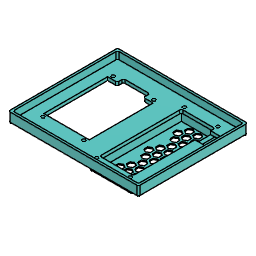
orient-beetle-screen-case-v2 v14 (Autodesk Fusion 360 design; units mm, degrees)
Autodesk Fusion 360 part; units mm, degrees
sketch "base-sketch" plane through (0, 0, 0) normal (0, 0, 1) x (1, 0, 0)
  line L0 (0, 0) -> (120, 0)
  line L1 (120, 0) -> (120, 100)
  line L2 (120, 100) -> (0, 100)
  line L3 (0, 100) -> (0, 0)
  line L4 (10, 19.5) -> (53.5, 19.5)
  line L5 (53.5, 19.5) -> (53.5, 80.5)
  line L6 (53.5, 80.5) -> (10, 80.5)
  line L7 (10, 80.5) -> (10, 19.5)
  line L8 (104, 11) -> (72, 11)
  line L9 (72, 11) -> (72, 89)
  line L10 (72, 89) -> (104, 89)
  line L11 (104, 89) -> (104, 11)
  line L12 (44.25, 86.5) -> (19.25, 86.5)
  line L13 (19.25, 86.5) -> (19.25, 80.5)
  line L14 (19.25, 80.5) -> (44.25, 80.5)
  line L15 (44.25, 80.5) -> (44.25, 86.5)
  line L16 (31.75, 19.5) -> (31.75, 80.5) construction
  line L17 (31.75, 80.5) -> (31.75, 86.5) construction
  line L18 (104, 70) -> (114, 70)
  line L19 (114, 70) -> (114, 85)
  line L20 (114, 85) -> (104, 85)
  line L21 (104, 85) -> (104, 70)
  circle A0 centre (116, 72.5) radius 1.25
  circle A1 centre (116, 82.5) radius 1.25
  line L22 (116, 72.5) -> (116, 82.5) construction
  line L23 (104, 77.5) -> (114, 77.5)
  circle A2 centre (12.25, 16.5) radius 1.6
  line L24 (10, 50) -> (53.5, 50) construction
  circle A3 centre (51.25, 16.5) radius 1.6
  circle A4 centre (12.25, 83.5) radius 1.6
  circle A5 centre (51.25, 83.5) radius 1.6
  line L25 (122.1, 102.1) -> (-2.1, 102.1)
  line L26 (-2.1, 102.1) -> (-2.1, -2.1)
  line L27 (-2.1, -2.1) -> (122.1, -2.1)
  line L28 (122.1, -2.1) -> (122.1, 102.1)
  point P0 (116, 77.5)
  dimension "d1" = 120
  dimension "d2" = 100
  dimension "d3" = 43.5
  dimension "d4" = 61
  dimension "d6" = 10
  dimension "d7" = 32
  dimension "d8" = 78
  dimension "d9" = 16
  dimension "d10" = 11
  dimension "d11" = 19.5
  dimension "d12" = 19.5
  dimension "d13" = 11
  dimension "d14" = 25
  dimension "d15" = 6
  dimension "d20" = 10
  dimension "d21" = 15
  dimension "d22" = 15
  dimension "d23" = 2.5
  dimension "d24" = 2.5
  dimension "d25" = 10
  dimension "d27" = 12
  dimension "d28" = 3.2
  dimension "d31" = 3.2
  dimension "d33" = 3.2
  dimension "d40" = 19.5
  dimension "d41" = 33.5
  dimension "d42" = 3.2
  dimension "d43" = 39
  dimension "d44" = 33.5
  dimension "d45" = 33.5
  dimension "d46" = 33.5
  dimension "d47" = 39
  dimension "d48" = 19.5
  dimension "d49" = 2.1
  constraint horizontal L0
  constraint vertical L1
  constraint horizontal L2
  constraint vertical L3
  constraint coincident L0.start L3.end
  constraint horizontal L4
  constraint vertical L5
  constraint horizontal L6
  constraint vertical L7
  constraint horizontal L8
  constraint vertical L9
  constraint horizontal L10
  constraint vertical L11
  constraint horizontal L12
  constraint vertical L13
  constraint horizontal L14
  constraint vertical L15
  constraint midpoint L4 L16.start
  constraint midpoint L6 L16.end
  constraint midpoint L14 L16.end
  constraint midpoint L12 L17.end
  constraint collinear L16 L17
  constraint collinear L6 L14
  constraint horizontal L18
  constraint vertical L19
  constraint horizontal L20
  constraint vertical L21
  constraint collinear L11 L21
  constraint coincident A0.centre L22.start
  constraint coincident A1.centre L22.end
  constraint parallel L19 L22
  constraint midpoint L21 L23.start
  constraint midpoint L19 L23.end
  constraint midpoint L22 P0
  constraint coincident L23 P0
  constraint midpoint L7 L24.start
  constraint midpoint L5 L24.end
  measures "d1" distance of L0.start L0.end
  measures "d2" distance of L0.start L2.end
  measures "d3" distance of L4.start L4.end
  measures "d4" distance of L4.start L6.end
  measures "d6" distance of L3 L7
  measures "d7" distance of L8.start L8.end
  measures "d8" distance of L8.start L10.end
  measures "d9" distance of L1 L11
  measures "d10" distance of L0 L8
  measures "d11" distance of L2 L6
  measures "d12" distance of L0 L4
  measures "d13" distance of L2 L10
  measures "d14" distance of L12.start L12.end
  measures "d15" distance of L12.end L13.end
  measures "d20" distance of L19.end L20.end
  measures "d21" distance of L18.end L19.end
  measures "d22" distance of L2 L20
  measures "d23" diameter of A0
  measures "d24" diameter of A1
  measures "d25" distance of A0.centre A1.centre
  measures "d27" distance of L21 A0.centre
  measures "d28" diameter of A2
  measures "d31" diameter of A3
  measures "d33" diameter of A4
  measures "d40" distance of L16 A4.centre
  measures "d41" distance of L24 A4.centre
  measures "d42" diameter of A5
  measures "d43" distance of A4.centre A5.centre
  measures "d44" distance of L24 A5.centre
  measures "d45" distance of A2.centre L24
  measures "d46" distance of L24 A3.centre
  measures "d47" distance of A2.centre A3.centre
  measures "d48" distance of L16 A2.centre
sketch "beetle-expansion" plane through (0, 0, 0) normal (0, 0, 1) x (1, 0, 0)
  line L0 (72, 89) -> (104, 89)
  line L1 (104, 89) -> (104, 11)
  line L2 (104, 11) -> (72, 11)
  line L3 (72, 11) -> (72, 89)
  line L4 (68, 7) -> (68, 93)
  line L5 (68, 93) -> (108, 93)
  line L6 (108, 93) -> (108, 7)
  line L7 (108, 7) -> (68, 7)
  dimension "d60" = -4
extrude "Extrude3" add sketch "beetle-expansion" against normal blind 8 makes body 1
sketch "beetle-expansion-top" plane through (0, 0, -8) normal (0, 0, -1) x (1, 0, 0)
  line L0 (72, -11) -> (104, -11)
  line L1 (104, -11) -> (104, -89)
  line L2 (104, -89) -> (72, -89)
  line L3 (72, -89) -> (72, -11)
  line L4 (108, -93) -> (108, -7)
  line L5 (108, -7) -> (68, -7)
  line L6 (68, -7) -> (68, -93)
  line L7 (68, -93) -> (108, -93)
  line L8 (104, -11) -> (104, -89)
  line L9 (72, -11) -> (104, -11)
  line L10 (72, -89) -> (72, -11)
  line L11 (104, -89) -> (72, -89)
extrude "Extrude1" add sketch "base-sketch" along normal blind 3.2 separate body contours L0 L1 L2 L3 makes body 2
extrude "Extrude2" add sketch "base-sketch" along normal blind 10 contours L25 L26 L27 L28 bodies 2
fillet "Fillet1" radius 1.5 8 edges at (-2.1, 102.1, 5) (122.1, 102.1, 5) (120, 0, 6.6) (-2.1, -2.1, 5) (0, 0, 6.6) (0, 100, 6.6) (120, 100, 6.6) (122.1, -2.1, 5) on bodies 2
fillet "Fillet2" radius 1.5 6 edges at (104, 11, 1.6) (72, 11, 1.6) (72, 89, 1.6) (104, 89, 1.6) (114, 70, 1.6) (114, 85, 1.6) on bodies 2
fillet "Fillet3" radius 1.5 2 edges at (44.25, 86.5, 1.6) (19.25, 86.5, 1.6) on bodies 2
extrude "Extrude6" add sketch "beetle-expansion-top" against normal blind 1 contours L0 L1 L2 L3 L8 L9 L10 L11 bodies 1
move_face "OffsetFaces1" offset 2 2 faces at (81.3333, 93, -5.3333) (94.6667, 7, -5.3333) on bodies 1
sketch "expansion-holes" plane through (0, 0, 3.2) normal (0, 0, 1) x (-1, 0, 0)
  line L0 (-44.25, -85) -> (-44.25, -80.5)
  line L1 (-44.25, -80.5) -> (-53.5, -80.5)
  line L2 (-53.5, -80.5) -> (-53.5, -19.5)
  line L3 (-53.5, -19.5) -> (-10, -19.5)
  line L4 (-10, -19.5) -> (-10, -80.5)
  line L5 (-10, -80.5) -> (-19.25, -80.5)
  line L6 (-19.25, -80.5) -> (-19.25, -85)
  arc A0 (-20.75, -86.5) -> (-19.25, -85) centre (-20.75, -85) ccw
  line L7 (-20.75, -86.5) -> (-42.75, -86.5)
  arc A1 (-44.25, -85) -> (-42.75, -86.5) centre (-42.75, -85) ccw
  line L8 (-112.5, -70) -> (-104, -70)
  line L9 (-104, -70) -> (-104, -12.5)
  arc A2 (-102.5, -11) -> (-104, -12.5) centre (-102.5, -12.5) ccw
  line L10 (-102.5, -11) -> (-73.5, -11)
  arc A3 (-72, -12.5) -> (-73.5, -11) centre (-73.5, -12.5) ccw
  line L11 (-72, -12.5) -> (-72, -87.5)
  arc A4 (-73.5, -89) -> (-72, -87.5) centre (-73.5, -87.5) ccw
  line L12 (-73.5, -89) -> (-102.5, -89)
  arc A5 (-104, -87.5) -> (-102.5, -89) centre (-102.5, -87.5) ccw
  line L13 (-104, -87.5) -> (-104, -85)
  line L14 (-104, -85) -> (-112.5, -85)
  arc A6 (-114, -83.5) -> (-112.5, -85) centre (-112.5, -83.5) ccw
  line L15 (-114, -83.5) -> (-114, -71.5)
  arc A7 (-112.5, -70) -> (-114, -71.5) centre (-112.5, -71.5) ccw
  circle A8 centre (-116, -82.5) radius 1.25
  circle A9 centre (-116, -72.5) radius 1.25
  circle A10 centre (-51.25, -83.5) radius 1.6
  circle A11 centre (-12.25, -83.5) radius 1.6
  circle A12 centre (-51.25, -16.5) radius 1.6
  circle A13 centre (-12.25, -16.5) radius 1.6
  arc A14 (-120, -98.5) -> (-118.5, -100) centre (-118.5, -98.5) ccw
  line L16 (-118.5, -100) -> (-1.5, -100)
  arc A15 (-1.5, -100) -> (0, -98.5) centre (-1.5, -98.5) ccw
  line L17 (0, -98.5) -> (0, -1.5)
  arc A16 (0, -1.5) -> (-1.5, 0) centre (-1.5, -1.5) ccw
  line L18 (-1.5, 0) -> (-118.5, 0)
  arc A17 (-118.5, 0) -> (-120, -1.5) centre (-118.5, -1.5) ccw
  line L19 (-120, -1.5) -> (-120, -98.5)
  circle A18 centre (-72, -92) radius 1.6
  line L20 (-68, -93) -> (-108, -93)
  line L21 (-68, -7) -> (-68, -93)
  line L22 (-72, -89) -> (-104, -89)
  dimension "d88" = 4
  dimension "d89" = 3.2
  dimension "d96" = 3
  measures "d88" distance of A18.centre L21
  measures "d89" diameter of A18
  measures "d96" distance of A18.centre L22
extrude "Extrude7" cut sketch "expansion-holes" against normal blind 15 contours A18 L20 | A18 L20 bodies 1 2
pattern_linear "R-Pattern1" count 2 spacing 32 along (1, 0, 0) count 2 spacing 84 along (0, -1, 0) of "Extrude7"
fillet "Fillet5" radius 1.5 4 edges at (68, 95, -4) (108, 95, -4) (68, 5, -4) (108, 5, -4) on bodies 1
sketch "honeycomb" plane through (0, 0, -8) normal (0, 0, -1) x (1, 0, 0)
  line L0 (104, -11) -> (72, -11) construction
  line L1 (72, -11) -> (72, -89) construction
  line L2 (104, -89) -> (104, -11) construction
  line L3 (72, -89) -> (104, -89) construction
  line L4 (104, -50) -> (72, -50) construction
  line L5 (88, -11) -> (88, -89) construction
  line L6 (88, -53.4641) -> (91, -51.7321)
  line L7 (91, -51.7321) -> (91, -48.2679)
  line L8 (91, -48.2679) -> (88, -46.5359)
  line L9 (88, -46.5359) -> (85, -48.2679)
  line L10 (85, -48.2679) -> (85, -51.7321)
  line L11 (85, -51.7321) -> (88, -53.4641)
  line L12 (88, -50) -> (86.5, -52.5981) construction
  line L13 (86.5, -52.5981) -> (86, -53.4641) construction
  line L14 (88, -50) -> (89.5, -52.5981) construction
  line L15 (84, -46.5359) -> (87, -44.8038)
  line L16 (87, -44.8038) -> (87, -41.3397)
  line L17 (87, -41.3397) -> (84, -39.6077)
  line L18 (84, -39.6077) -> (81, -41.3397)
  line L19 (81, -44.8038) -> (84, -46.5359)
  line L20 (81, -41.3397) -> (81, -44.8038)
  line L21 (80, -53.4641) -> (83, -51.7321)
  line L22 (83, -51.7321) -> (83, -48.2679)
  line L23 (83, -48.2679) -> (80, -46.5359)
  line L24 (80, -46.5359) -> (77, -48.2679)
  line L25 (77, -51.7321) -> (80, -53.4641)
  line L26 (77, -48.2679) -> (77, -51.7321)
  line L27 (92, -46.5359) -> (95, -44.8038)
  line L28 (95, -44.8038) -> (95, -41.3397)
  line L29 (95, -41.3397) -> (92, -39.6077)
  line L30 (92, -39.6077) -> (89, -41.3397)
  line L31 (89, -44.8038) -> (92, -46.5359)
  line L32 (89, -41.3397) -> (89, -44.8038)
  line L33 (84, -60.3923) -> (87, -58.6603)
  line L34 (87, -58.6603) -> (87, -55.1962)
  line L35 (87, -55.1962) -> (84, -53.4641)
  line L36 (84, -53.4641) -> (81, -55.1962)
  line L37 (81, -58.6603) -> (84, -60.3923)
  line L38 (81, -55.1962) -> (81, -58.6603)
  line L39 (96, -53.4641) -> (99, -51.7321)
  line L40 (99, -51.7321) -> (99, -48.2679)
  line L41 (99, -48.2679) -> (96, -46.5359)
  line L42 (96, -46.5359) -> (93, -48.2679)
  line L43 (93, -51.7321) -> (96, -53.4641)
  line L44 (93, -48.2679) -> (93, -51.7321)
  line L45 (92, -60.3923) -> (95, -58.6603)
  line L46 (95, -58.6603) -> (95, -55.1962)
  line L47 (95, -55.1962) -> (92, -53.4641)
  line L48 (92, -53.4641) -> (89, -55.1962)
  line L49 (89, -58.6603) -> (92, -60.3923)
  line L50 (89, -55.1962) -> (89, -58.6603)
  line L51 (87, -27.4962) -> (84, -25.7641)
  line L52 (84, -25.7641) -> (81, -27.4962)
  line L53 (81, -27.4962) -> (81, -30.9603)
  line L54 (81, -30.9603) -> (84, -32.6923)
  line L55 (87, -30.9603) -> (87, -27.4962)
  line L56 (84, -32.6923) -> (87, -30.9603)
  line L57 (95, -27.4962) -> (92, -25.7641)
  line L58 (92, -25.7641) -> (89, -27.4962)
  line L59 (89, -27.4962) -> (89, -30.9603)
  line L60 (89, -30.9603) -> (92, -32.6923)
  line L61 (95, -30.9603) -> (95, -27.4962)
  line L62 (92, -32.6923) -> (95, -30.9603)
  line L63 (99, -20.5679) -> (96, -18.8359)
  line L64 (96, -18.8359) -> (93, -20.5679)
  line L65 (93, -20.5679) -> (93, -24.0321)
  line L66 (93, -24.0321) -> (96, -25.7641)
  line L67 (99, -24.0321) -> (99, -20.5679)
  line L68 (96, -25.7641) -> (99, -24.0321)
  line L69 (95, -13.6397) -> (92, -11.9077)
  line L70 (92, -11.9077) -> (89, -13.6397)
  line L71 (89, -13.6397) -> (89, -17.1038)
  line L72 (89, -17.1038) -> (92, -18.8359)
  line L73 (95, -17.1038) -> (95, -13.6397)
  line L74 (92, -18.8359) -> (95, -17.1038)
  line L75 (81, -13.6397) -> (81, -17.1038)
  line L76 (81, -17.1038) -> (84, -18.8359)
  line L77 (84, -18.8359) -> (87, -17.1038)
  line L78 (87, -17.1038) -> (87, -13.6397)
  line L79 (84, -11.9077) -> (81, -13.6397)
  line L80 (87, -13.6397) -> (84, -11.9077)
  line L81 (77, -20.5679) -> (77, -24.0321)
  line L82 (77, -24.0321) -> (80, -25.7641)
  line L83 (80, -25.7641) -> (83, -24.0321)
  line L84 (83, -24.0321) -> (83, -20.5679)
  line L85 (80, -18.8359) -> (77, -20.5679)
  line L86 (83, -20.5679) -> (80, -18.8359)
  line L87 (85, -24.0321) -> (88, -25.7641)
  line L88 (88, -25.7641) -> (91, -24.0321)
  line L89 (91, -24.0321) -> (91, -20.5679)
  line L90 (91, -20.5679) -> (88, -18.8359)
  line L91 (85, -20.5679) -> (85, -24.0321)
  line L92 (88, -18.8359) -> (85, -20.5679)
  line L93 (87, -82.8962) -> (84, -81.1641)
  line L94 (84, -81.1641) -> (81, -82.8962)
  line L95 (81, -82.8962) -> (81, -86.3603)
  line L96 (81, -86.3603) -> (84, -88.0923)
  line L97 (87, -86.3603) -> (87, -82.8962)
  line L98 (84, -88.0923) -> (87, -86.3603)
  line L99 (95, -82.8962) -> (92, -81.1641)
  line L100 (92, -81.1641) -> (89, -82.8962)
  line L101 (89, -82.8962) -> (89, -86.3603)
  line L102 (89, -86.3603) -> (92, -88.0923)
  line L103 (95, -86.3603) -> (95, -82.8962)
  line L104 (92, -88.0923) -> (95, -86.3603)
  line L105 (99, -75.9679) -> (96, -74.2359)
  line L106 (96, -74.2359) -> (93, -75.9679)
  line L107 (93, -75.9679) -> (93, -79.4321)
  line L108 (93, -79.4321) -> (96, -81.1641)
  line L109 (99, -79.4321) -> (99, -75.9679)
  line L110 (96, -81.1641) -> (99, -79.4321)
  line L111 (95, -69.0397) -> (92, -67.3077)
  line L112 (92, -67.3077) -> (89, -69.0397)
  line L113 (89, -69.0397) -> (89, -72.5038)
  line L114 (89, -72.5038) -> (92, -74.2359)
  line L115 (95, -72.5038) -> (95, -69.0397)
  line L116 (92, -74.2359) -> (95, -72.5038)
  line L117 (81, -69.0397) -> (81, -72.5038)
  line L118 (81, -72.5038) -> (84, -74.2359)
  line L119 (84, -74.2359) -> (87, -72.5038)
  line L120 (87, -72.5038) -> (87, -69.0397)
  line L121 (84, -67.3077) -> (81, -69.0397)
  line L122 (87, -69.0397) -> (84, -67.3077)
  line L123 (77, -75.9679) -> (77, -79.4321)
  line L124 (77, -79.4321) -> (80, -81.1641)
  line L125 (80, -81.1641) -> (83, -79.4321)
  line L126 (83, -79.4321) -> (83, -75.9679)
  line L127 (80, -74.2359) -> (77, -75.9679)
  line L128 (83, -75.9679) -> (80, -74.2359)
  line L129 (85, -79.4321) -> (88, -81.1641)
  line L130 (88, -81.1641) -> (91, -79.4321)
  line L131 (91, -79.4321) -> (91, -75.9679)
  line L132 (91, -75.9679) -> (88, -74.2359)
  line L133 (85, -75.9679) -> (85, -79.4321)
  line L134 (88, -74.2359) -> (85, -75.9679)
  line L135 (91, -37.8771) -> (91, -34.4129)
  line L136 (91, -34.4129) -> (88, -32.6809)
  line L137 (88, -32.6809) -> (85, -34.4129)
  line L138 (85, -34.4129) -> (85, -37.8771)
  line L139 (88, -39.6091) -> (91, -37.8771)
  line L140 (85, -37.8771) -> (88, -39.6091)
  line L141 (91, -65.5871) -> (91, -62.1229)
  line L142 (91, -62.1229) -> (88, -60.3909)
  line L143 (88, -60.3909) -> (85, -62.1229)
  line L144 (85, -62.1229) -> (85, -65.5871)
  line L145 (88, -67.3191) -> (91, -65.5871)
  line L146 (85, -65.5871) -> (88, -67.3191)
  point P0 (88, -50)
  point P1 (88, -50)
  dimension "d122" = 60
  dimension "d124" = 1
  dimension "d125" = 3
  dimension "d128" = 8
  dimension "d129" = 8
  dimension "d134" = 27.7
  dimension "d135" = 0
  dimension "d138" = 13.855
  dimension "d139" = 0
  constraint midpoint L2 L4.start
  constraint midpoint L1 L4.end
  constraint midpoint L0 L5.start
  constraint midpoint L3 L5.end
  constraint midpoint L5 P1
  constraint coincident P1 P0
  constraint midpoint L11 L12.end
  constraint perpendicular L11 L13
  constraint midpoint L6 L14.end
  measures "d122" angle of L1 L11
  measures "d124" distance of L12.end L13.end
  measures "d125" distance of P1 L11
extrude "Extrude9" cut sketch "honeycomb" against normal blind 10 bodies 1
fillet "Fillet6" radius 1.5 8 edges at (107.5607, 94.5607, -8) (108, 50, -8) (107.5607, 5.4393, -8) (88, 5, -8) (68.4393, 5.4393, -8) (68, 50, -8) (68.4393, 94.5607, -8) (88, 95, -8) on bodies 1
fillet "Fillet7" radius 1.5 8 edges at (-2.1, 50, 0) (-1.6607, -1.6607, 0) (60, -2.1, 0) (121.6607, -1.6607, 0) (122.1, 50, 0) (121.6607, 101.6607, 0) (60, 102.1, 0) (-1.6607, 101.6607, 0) on bodies 2
fillet "Fillet8" radius 1.5 2 edges at (44.25, 80.5, 1.6) (19.25, 80.5, 1.6) on bodies 2
named bodies: "main-case-body", "beetle-expansion"
